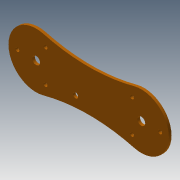
# Autodesk Inventor part: dibond_strana(b1)
Saved by Autodesk Inventor 2013 (Build 170138000, 138)
## iProperties
Created: 2013-05-11
Part Number: dibond_strana(b1)
Material: Generic
Document SubType Name: Modeling
Designer: idle-rug
Density: 1 g/cm^3
Author: idle-rug
Autodesk Inventor part; units mm, degrees
ref_plane "YZ Plane" through (0, 0, 0) normal (1, 0, 0) x (0, 1, 0)
ref_plane "XZ Plane" through (0, 0, 0) normal (0, 1, 0) x (-1, 0, 0)
ref_plane "XY Plane" through (0, 0, 0) normal (0, 0, 1) x (1, 0, 0)
sketch "Sketch1" plane through (0, 0, 0) normal (0, 1, 0) x (-1, 0, 0)
  line L0 (-50.5, -21) -> (-38.580998, -21)
  line L1 (-50.5, -21) -> (-38.580998, -21)
  line L2 (-50.5, 21) -> (-38.580998, 21)
  arc A0 (-50.5, 21) -> (-50.5, -21) centre (-50.5, 0) ccw
  circle A1 centre (40, 0) radius 3
  line L3 (-71.5, 0) -> (-61.5, 0)
  line L4 (-50.5, 21) -> (-37.146287, 21)
  arc A2 (-37.146287, 21) -> (34.589084, 20.290934) centre (0, 150) ccw
  line L5 (-50.5, -21) -> (-37.146287, -21)
  arc A3 (34.589084, -20.290934) -> (-37.146287, -21) centre (0, -150) ccw
  circle A4 centre (-61.5, 0) radius 2
  line L6 (40, 0) -> (20, 0)
  circle A5 centre (20, 0) radius 2
  arc A6 (37.224562, -20.815786) -> (37.224562, 20.815786) centre (40, 0) ccw
  arc A7 (34.589084, -20.290934) -> (34.589084, 20.290934) centre (40, 0) ccw
  point P0 (0, 0)
  point P1 (0, 0)
  dimension "d1" = 6
  dimension "d3" = 10
  dimension "d5" = 4
  dimension "d7" = 4
  constraints: 14 end point, 11 point on circle, 8 centre point, 5 tangent, 2 coincident, 1 point on line
  measures "d1" diameter of A1
  measures "d3" distance of L3.start L3.end
  measures "d5" diameter of A4
  measures "d7" diameter of A5
extrude "Extrusion1" add sketch "Sketch1" along normal blind 2
sketch "Sketch2" plane through (0, 2, 0) normal (0, 1, 0) x (1, 0, 0)
  circle A0 centre (-54.25, 0) radius 1.5
  circle A1 centre (-32.875, 12.340862) radius 1.5
  circle A2 centre (-32.875, -12.340862) radius 1.5
  point P0 (0, 0)
  dimension "d11" = 3
  dimension "d14" = 3
  dimension "d15" = 3
  constraints: 3 centre point
  measures "d11" diameter of A0
  measures "d14" diameter of A1
  measures "d15" diameter of A2
extrude "Extrusion2" cut sketch "Sketch2" against normal blind 2
sketch "Sketch3" plane through (0, 2, 0) normal (0, 1, 0) x (1, 0, 0)
  line L0 (37.146287, -21) -> (50.5, -21)
  arc A0 (50.5, -21) -> (50.5, 21) centre (50.5, 0) ccw
  line L1 (50.5, 0) -> (40, 0)
  circle A1 centre (40, 0) radius 3
  point P0 (0, 0)
  dimension "d18" = 10.5
  dimension "d19" = 6
  constraints: 2 end point, 1 centre point, 1 coincident, 1 parallel
  measures "d18" distance of L1.start L1.end
  measures "d19" diameter of A1
extrude "Extrusion3" cut sketch "Sketch3" against normal blind 2
sketch "Sketch4" plane through (0, 0, 0) normal (0, -1, 0) x (1, 0, 0)
  circle A0 centre (40, 0) radius 3
  line L0 (40, 0) -> (54.25, 0) construction
  line L1 (40, 0) -> (54.25, 0) construction
  line L2 (40, 0) -> (54.25, 0) construction
  line L3 (40, 0) -> (54.25, 0) construction
  circle A1 centre (47.125, 12.340862) radius 1.5
  circle A2 centre (25.75, 0) radius 1.5
  circle A3 centre (47.125, -12.340862) radius 1.5
  point P0 (0, 0)
  dimension "d33" = 3
  dimension "d34" = 3
  dimension "d35" = 3
  constraints: 8 end point, 4 horizontal, 3 centre point, 1 coincident
  measures "d33" diameter of A1
  measures "d34" diameter of A2
  measures "d35" diameter of A3
extrude "Extrusion4" cut sketch "Sketch4" against normal blind 2 contours A1 | A2 | A3
sketch "Sketch5" plane through (0, 0, 0) normal (0, -1, 0) x (1, 0, 0)
  circle A0 centre (25.75, 0) radius 1.5
  circle A1 centre (47.125, 12.340862) radius 1.5
  circle A2 centre (47.125, -12.340862) radius 1.5
  circle A3 centre (40, 0) radius 3
  arc A4 (-34.589084, 20.290934) -> (37.146287, 21) centre (0, 150) ccw
  circle A5 centre (40, 0) radius 21
  point P0 (0, 0)
  constraints: 1 centre point, 1 coincident, 1 tangent
extrude "Extrusion5" cut sketch "Sketch5" against normal blind 10
sketch "Sketch6" plane through (0, 0, 0) normal (0, -1, 0) x (1, 0, 0)
  arc A0 (40, 21) -> (34.589084, 20.290934) centre (40, 0) ccw
  line L0 (37.146287, 21) -> (40, 21)
  arc A1 (34.589084, 20.290934) -> (37.146287, 21) centre (0, 150) ccw
  point P0 (0, 0)
extrude "Extrusion6" cut sketch "Sketch6" against normal blind 2
sketch "Sketch7" plane through (0, 0, 0) normal (0, -1, 0) x (1, 0, 0)
  arc A0 (60.912791, 1.911854) -> (40, 21) centre (40, 0) ccw
  arc A1 (60.912791, -1.911854) -> (60.912791, 1.911854) centre (61.5, 0) ccw
  arc A2 (40, -21) -> (60.912791, -1.911854) centre (40, 0) ccw
  line L0 (50.5, -21) -> (40, -21)
  arc A3 (50.5, -21) -> (50.5, 21) centre (50.5, 0) ccw
  line L1 (40, 21) -> (50.5, 21)
  point P0 (0, 0)
extrude "Extrusion7" cut sketch "Sketch7" against normal blind 2
sketch "Sketch8" plane through (0, 0, 0) normal (0, -1, 0) x (1, 0, 0)
  arc A0 (34.589084, -20.290934) -> (40, -21) centre (40, 0) ccw
  arc A1 (37.146287, -21) -> (34.589084, -20.290934) centre (0, -150) ccw
  line L0 (40, -21) -> (37.146287, -21)
  point P0 (0, 0)
extrude "Extrusion8" cut sketch "Sketch8" against normal blind 2
sketch "Sketch9" plane through (0, 0, 0) normal (0, -1, 0) x (1, 0, 0)
  arc A0 (34.589084, 20.290934) -> (34.589084, -20.290934) centre (40, 0) ccw
  circle A1 centre (40, 0) radius 21
  circle A2 centre (40, 0) radius 3
  circle A3 centre (54.25, 0) radius 1.5
  line L0 (40, 0) -> (32.875, 12.340862)
  line L1 (40, 0) -> (54.25, 0) construction
  line L2 (40, 0) -> (32.875, -12.340862)
  line L3 (40, 0) -> (54.25, 0) construction
  circle A4 centre (32.875, 12.340862) radius 1.5
  circle A5 centre (32.875, -12.340862) radius 1.5
  point P0 (0, 0)
  dimension "d47" = 6
  dimension "d48" = 3
  dimension "d49" = 120
  dimension "d50" = 120
  dimension "d51" = 3
  dimension "d52" = 3
  constraints: 8 end point, 5 centre point, 3 coincident, 2 equal length, 2 horizontal, 1 concentric
  measures "d47" diameter of A2
  measures "d48" diameter of A3
  measures "d49" angle of L1 L0
  measures "d50" angle of L2 L3
  measures "d51" diameter of A4
  measures "d52" diameter of A5
extrude "Extrusion9" add sketch "Sketch9" against normal blind 2
sketch "Sketch10" plane through (0, 0, 0) normal (0, -1, 0) x (1, 0, 0)
  circle A0 centre (-20, 0) radius 2
  arc A1 (-34.589084, 20.290934) -> (34.589084, 20.290934) centre (0, 150) ccw
  arc A2 (-34.589084, 20.290934) -> (-34.589084, -20.290934) centre (-40, 0) ccw
  line L0 (-40, 0) -> (-10, 0)
  line L1 (-10, 0) -> (-10, 16.131234)
  line L2 (-10, 0) -> (-10, 8)
  circle A3 centre (-10, 8) radius 2
  point P0 (0, 0)
  dimension "d55" = 30
  dimension "d56" = 8
  dimension "d57" = 4
  constraints: 6 end point, 1 centre point, 1 coincident, 1 horizontal, 1 perpendicular, 1 point on circle, 1 point on line
  measures "d55" distance of L0.start L0.end
  measures "d56" distance of L0.end L2.end
  measures "d57" diameter of A3
extrude "Extrusion10" add sketch "Sketch10" against normal blind 2
sketch "Sketch11" plane through (0, 0, 0) normal (0, -1, 0) x (1, 0, 0)
  circle A0 centre (-10, -8) radius 2
  point P0 (0, 0)
  dimension "d63" = 4
  constraints: 1 centre point
  measures "d63" diameter of A0
extrude "Extrusion11" cut sketch "Sketch11" against normal blind 2
body "Solid1"
